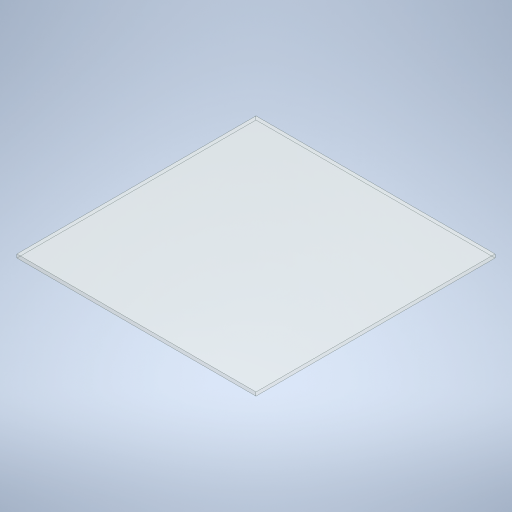
# Autodesk Inventor part: Topbottom
Saved by Autodesk Inventor 2024 (Build 280153000, 153)
## iProperties
Created: 2023-05-31
Part Number: Topbottom
Material: Glass
Document SubType Name: Modeling
Designer: shrus
Density: 2.18 g/cm^3
Appearance: Clear
Author: shrus
Autodesk Inventor part; units mm, degrees
ref_plane "YZ Plane" through (0, 0, 0) normal (1, 0, 0) x (0, 1, 0)
ref_plane "XZ Plane" through (0, 0, 0) normal (0, 1, 0) x (-1, 0, 0)
ref_plane "XY Plane" through (0, 0, 0) normal (0, 0, 1) x (1, 0, 0)
sketch "Sketch1" plane through (0, 0, 0) normal (0, 1, 0) x (-1, 0, 0)
  line L0 (11.5111, 11.0922) -> (11.5111, -188.9078)
  line L1 (11.5111, -188.9078) -> (-188.4889, -188.9078)
  line L2 (-188.4889, -188.9078) -> (-188.4889, 11.0922)
  line L3 (-188.4889, 11.0922) -> (11.5111, 11.0922)
  point P0 (0, 0)
  dimension "d0" = 200
  dimension "d1" = 200
  constraints: 8 end point, 2 perpendicular, 1 horizontal, 1 vertical
  measures "d0" distance of L0.start L0.end
  measures "d1" distance of L0.end L1.end
extrude "Extrusion1" add sketch "Sketch1" along normal blind 3
body "Solid1"
